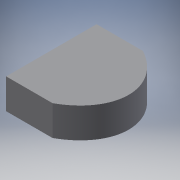
# Autodesk Inventor part: Intersect
Saved by Autodesk Inventor 2018 (Build 220112000, 112)
## iProperties
Created: 2005-07-19
Part Number: Intersect
Document SubType Name: Modeling
Designer: Administrator
Manufacturer: Standard
Standards Organization: Custom
Material: Generic
Density: 1 g/cm^3
Appearance: Default
Author: Administrator
Autodesk Inventor part; units mm, degrees
ref_plane "YZ Plane" through (0, 0, 0) normal (1, 0, 0) x (0, 1, 0)
ref_plane "XZ Plane" through (0, 0, 0) normal (0, 1, 0) x (-1, 0, 0)
ref_plane "XY Plane" through (0, 0, 0) normal (0, 0, 1) x (1, 0, 0)
sketch "Sketch1" plane through (0, 0, 0) normal (0, 0, 1) x (1, 0, 0)
  line L0 (-28.575, 14.2875) -> (47.625, 14.2875)
  line L1 (47.625, 14.2875) -> (47.625, -61.9125)
  line L2 (47.625, -61.9125) -> (-28.575, -61.9125)
  line L3 (-28.575, -61.9125) -> (-28.575, 14.2875)
  dimension "d0" = 76.2
  dimension "d1" = 76.2
  constraints: 8 end point, 2 parallel, 1 horizontal, 1 perpendicular
  measures "d0" distance of L0.start L0.end
  measures "d1" distance of L2.end L0.start
extrude "Extrusion1" add sketch "Sketch1" along normal blind 76.2
sketch "Sketch2" plane through (-28.575, 14.2875, 0) normal (0, 1, 0) x (1, 0, 0)
  line L0 (0, 0) -> (0, -76.2) projected
  ellipse E0 centre (0, -38.1) end of major axis (0, -85.725) minor radius 65.1237
  constraints: 1 midpoint, 2 other
extrude "Extrusion3" cut sketch "Sketch2" against normal blind 25.4 keep common part
body "Solid1"
